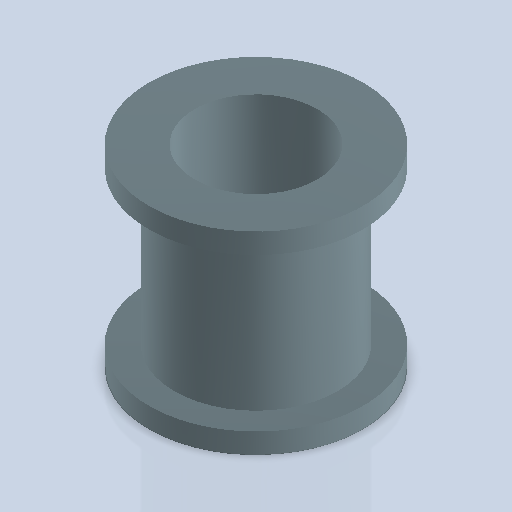
# Autodesk Inventor part: 2033
Saved by Autodesk Inventor 2024 (Build 280153000, 153)
## iProperties
Created: 2024-06-11
Part Number: 2033
Material: Blei
Document SubType Name: Modeling
Designer: ffogue
Density: 11.34 g/cm^3
Appearance: Blei
Author: ffogue
Autodesk Inventor part; units mm, degrees
ref_plane "YZ Plane" through (0, 0, 0) normal (1, 0, 0) x (0, 1, 0)
ref_plane "XY Plane" through (0, 0, 0) normal (0, 0, 1) x (1, 0, 0)
sketch "Skizze1" plane through (0, 0, 0) normal (0, 1, 0) x (-1, 0, 0)
  line L0 (0, 0) -> (10.5, 0)
  line L1 (10.5, 0) -> (10.5, -2)
  line L2 (10.5, -2) -> (8, -2)
  line L3 (8, -2) -> (8, -17)
  line L4 (8, -17) -> (10.5, -17)
  line L5 (10.5, -17) -> (10.5, -19)
  line L6 (10.5, -19) -> (0, -19)
  line L7 (0, -19) -> (0, 0)
  point P0 (0, -9.5)
  dimension "d0" = 2
  dimension "d1" = 2
  dimension "d2" = 21
  dimension "d3" = 16
  dimension "d4" = 19
  constraints: 16 end point, 6 perpendicular, 2 point on line, 1 horizontal, 1 midpoint
  measures "d0" distance between parallel lines of L2 L0
  measures "d1" distance between parallel lines of L6 L4
  measures "d2" diameter of L1 L7
  measures "d3" diameter of L3 point (0, -9.5)
  measures "d4" distance between parallel lines of L6 L0
revolve "Umdrehung1" add sketch "Skizze1" angle 360 about axis through (0, 0, -19) along (0, 0, 1)
sketch "Skizze2" plane through (0, 0, 0) normal (0, 0, 1) x (1, 0, 0)
  circle A0 centre (0, 0) radius 10.5 projected
  point P0 (0, 0)
  constraints: 1 coincident
hole "Bohrung1" at (0, 0, 0) direction (0, 0, -1) diameter 12 end through all
ref_plane "Arbeitsebene1" through (0, 8, 0) normal (0, 1, 0) x (-1, 0, 0)
sketch "Skizze3" plane through (0, 8, 0) normal (0, 1, 0) x (-1, 0, 0)
  line L0 (10.5, 0) -> (-10.5, 0) projected
  point P0 (0, 0)
  point P1 (0, -9.5)
  point P2 (0, 0)
  dimension "d14" = 9.5
  constraints: 1 midpoint, 1 vertical alignment
  measures "d14" distance from line of L0 point (0, -9.5)
hole "Bohrung2" at (0, 8, -9.5) direction (0, -1, 0) diameter 3 depth 5
equation "\"d1\" = d0"
